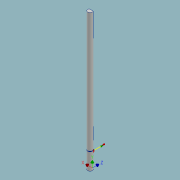
# Autodesk Inventor part: AA054
Saved by Autodesk Inventor 2017 SP1 (Build 210196100, 196)
## iProperties
Created: 2018-06-21
Part Number: AA054
Material: Aluminum 6061
Document SubType Name: Modeling
Designer: Zach
Density: 2.7 g/cm^3
Appearance: Aluminum - Flat
Author: Zach
Autodesk Inventor part; units mm, degrees
ref_plane "YZ Plane" through (0, 0, 0) normal (1, 0, 0) x (0, 1, 0)
ref_plane "XZ Plane" through (0, 0, 0) normal (0, 1, 0) x (-1, 0, 0)
sketch "Sketch1" plane through (0, 0, 0) normal (0, 0, 1) x (1, 0, 0)
  circle A0 centre (0, 0) radius 4
  dimension "d0" = 8
  constraints: 1 centre point, 1 coincident
  measures "d0" diameter of A0
extrude "Extrusion1" add sketch "Sketch1" along normal blind 235
sketch "Sketch5" plane through (0, 0, 235) normal (0, 0, 1) x (1, 0, 0)
  circle A0 centre (0, 0) radius 4 projected
  line L0 (-3.4641, 2) -> (3.4641, 2)
  arc A1 (3.4641, 2) -> (-3.4641, 2) centre (0, 0) ccw
  dimension "d18" = 2
  constraints: 4 point on circle, 2 end point, 1 centre point, 1 concentric, 1 horizontal
  measures "d18" distance from line of point (0, 0) L0
extrude "Extrusion5" cut sketch "Sketch5" against normal blind 40 contours L0 A0 picked at (-0.1548, 2.6577)
sketch "Sketch7" plane through (-3.4641, 2, 235) normal (0, 1, 0) x (1, 0, 0)
  circle A0 centre (3.4641, 209.45) radius 1.5
  circle A1 centre (3.4641, 212.2) radius 1.5
  line L0 (1.9641, 209.45) -> (1.9641, 212.2)
  line L1 (4.9641, 209.45) -> (4.9641, 212.2)
  line L2 (-0.5359, 235) -> (-0.5359, 0) projected
  line L3 (7.4641, 235) -> (7.4641, 0) projected
  line L4 (-0.5359, 191) -> (7.4641, 191)
  line L5 (7.4641, 191) -> (7.4641, 171)
  line L6 (7.4641, 171) -> (-0.5359, 171)
  line L7 (-0.5359, 171) -> (-0.5359, 191)
  point P0 (3.4641, 235)
  dimension "d21" = 3
  dimension "d22" = 3
  dimension "d23" = 2.75
  dimension "d24" = 22.8
  dimension "d25" = 20
  dimension "d26" = 44
  constraints: 12 end point, 4 point on circle, 4 tangent, 2 centre point, 2 parallel, 2 point on line, 2 vertical alignment, 1 horizontal, 1 perpendicular
  measures "d21" diameter of A0
  measures "d22" diameter of A1
  measures "d23" distance of A0.centre A1.centre
  measures "d24" distance of point (3.464, 235) A1.centre
  measures "d25" distance between parallel lines of L4 L6
  measures "d26" distance from line of point (3.464, 235) L4
extrude "Extrusion6" cut sketch "Sketch7" along normal through all
ref_plane "Work Plane1" through (0, 0, 28.55) normal (0, 0, -1) x (-1, 0, 0)
sketch "Sketch8" plane through (0, 0, 28.55) normal (0, 0, -1) x (-1, 0, 0)
  circle A0 centre (0, 0) radius 4 projected
  circle A1 centre (0, 0) radius 3.2
  dimension "d30" = 0.8
  constraints: 1 centre point
  measures "d30" radial gap between concentric circles of A0 A1
extrude "Extrusion7" cut sketch "Sketch8" against normal blind 1
body "Solid1"
